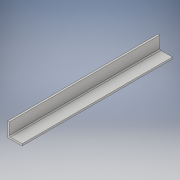
# Autodesk Inventor part: uchannel
Saved by Autodesk Inventor 2017 (Build 210142000, 142)
## iProperties
Created: 2018-10-17
Part Number: uchannel
Material: Generic
Document SubType Name: Modeling
Designer: ddeboer
Density: 1 g/cm^3
Appearance: Default
Author: ddeboer
Autodesk Inventor part; units mm, degrees
ref_plane "YZ Plane" through (0, 0, 0) normal (1, 0, 0) x (0, 1, 0)
ref_plane "XZ Plane" through (0, 0, 0) normal (0, 1, 0) x (-1, 0, 0)
ref_plane "XY Plane" through (0, 0, 0) normal (0, 0, 1) x (1, 0, 0)
sketch "Sketch1" plane through (0, 0, 0) normal (0, 0, 1) x (1, 0, 0)
  arc A0 (3.175, 4.953) -> (4.953, 3.175) centre (4.953, 4.953) ccw
  line L0 (0, 0) -> (25.4, 0)
  line L1 (0, 0) -> (0, 25.4)
  line L2 (3.175, 4.953) -> (3.175, 25.4)
  line L3 (3.175, 25.4) -> (0, 25.4)
  line L4 (4.953, 3.175) -> (25.4, 3.175)
  line L5 (25.4, 3.175) -> (25.4, 0)
  dimension "d6" = 25.4
  dimension "d7" = 25.4
  constraints: 12 end point, 2 horizontal, 2 perpendicular, 2 point on circle, 2 vertical, 1 centre point
  measures "d6" distance of L0.start L0.end
  measures "d7" distance of L0.start L1.end
extrude "Extrusion1" add sketch "Sketch1" along normal blind 263.525
body "Solid1"
